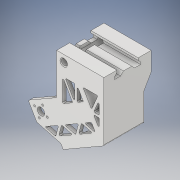
# Autodesk Inventor part: Gantry_Mount
Saved by Autodesk Inventor 2019 (Build 230136000, 136)
## iProperties
Created: 2021-01-31
Part Number: Gantry_Mount
Material: ABS Plastic
Document SubType Name: Modeling
Designer: zhanb
Density: 1.06 g/cm^3
Appearance: Smooth - White
Author: zhanb
Autodesk Inventor part; units mm, degrees
ref_plane "YZ Plane" through (0, 0, 0) normal (1, 0, 0) x (0, 1, 0)
ref_plane "XZ Plane" through (0, 0, 0) normal (0, 1, 0) x (-1, 0, 0)
ref_plane "XY Plane" through (0, 0, 0) normal (0, 0, 1) x (1, 0, 0)
sketch "Sketch1" plane through (0, 0, 0) normal (0, 0, 1) x (1, 0, 0)
  line L0 (-25.4, -44.45) -> (-18.594091, -44.45)
  line L1 (25.4, -44.45) -> (25.4, -19.05) construction
  line L2 (25.4, 44.45) -> (-25.4, 44.45)
  line L3 (-25.4, 44.45) -> (-25.4, -42.513515)
  line L4 (-25.4, -44.45) -> (25.4, 44.45) construction
  line L5 (25.4, -44.45) -> (-25.4, 44.45) construction
  line L6 (-18.594091, -44.45) -> (25.4, -19.05)
  line L7 (-18.594091, -44.45) -> (-35.091874, -53.975) construction
  line L8 (-35.091874, -53.975) -> (-37.631874, -49.575591) construction
  line L9 (-37.631874, -49.575591) -> (-25.4, -42.513515) construction
  line L10 (-21.134091, -40.050591) -> (-18.594091, -44.45) construction
  line L11 (-18.594091, -44.45) -> (25.4, -44.45) construction
  line L12 (-25.4, -42.513515) -> (-25.4, -44.45)
  line L13 (-25.4, -42.513515) -> (-21.134091, -40.050591) construction
  line L14 (25.4, -19.05) -> (25.4, 44.45)
  point P0 (0, 0)
  dimension "d0" = 30
  dimension "d1" = 50.8
  dimension "d2" = 88.9
  dimension "d3" = 50.8
  dimension "d4" = 5.08
  dimension "d5" = 19.05
  constraints: 30 end point, 9 parallel, 5 perpendicular, 2 horizontal, 2 midpoint, 1 point on line
  measures "d0" angle of L0 L6
  measures "d1" distance of L0.end L1.end
  measures "d2" distance of L2.end L0.start
  measures "d3" distance of L2.start L2.end
  measures "d4" distance of L7.end L8.end
  measures "d5" distance of L0.end L7.end
extrude "Extrusion1" add sketch "Sketch1" along normal mid plane 50.8
sketch "Sketch5" plane through (-25.4, -42.513515, 25.4) normal (-1, 0, 0) x (0, 0, 1)
  line L0 (0, 86.963515) -> (0, -1.936485) construction
  line L1 (-50.8, 86.963515) -> (0, 86.963515) construction
  line L2 (-50.8, -1.936485) -> (-50.8, 86.963515) construction
  line L3 (-36.83, 86.963515) -> (-36.83, 84.621952)
  line L4 (-36.83, 84.621952) -> (-39.37, 82.081952)
  line L5 (-39.37, 82.081952) -> (-39.37, 79.541952)
  line L6 (-39.37, 79.541952) -> (-33.02, 79.541952)
  line L7 (-33.02, 79.541952) -> (-29.845, 82.716952)
  line L8 (-29.845, 82.716952) -> (-20.955, 82.716952)
  line L9 (-20.955, 82.716952) -> (-17.78, 79.541952)
  line L10 (-17.78, 79.541952) -> (-11.43, 79.541952)
  line L11 (-11.43, 79.541952) -> (-11.43, 82.081952)
  line L12 (-11.43, 82.081952) -> (-13.97, 84.621952)
  line L13 (-13.97, 84.621952) -> (-13.97, 86.963515)
  line L14 (-25.4, 42.513515) -> (-25.4, 86.963515) construction
  line L15 (-36.83, 86.963515) -> (-13.97, 86.963515)
  line L16 (0, -1.936485) -> (-50.8, -1.936485)
  point P0 (-25.4, 42.513515)
  dimension "d22" = 135
  dimension "d23" = 11.43
  dimension "d24" = 2.34156
  dimension "d25" = 2.54
  dimension "d26" = 3.175
  dimension "d27" = 13.97
  dimension "d28" = 6.35
  constraints: 26 end point, 4 parallel, 4 point on line, 2 perpendicular, 1 coincident, 1 collinear, 1 midpoint, 5 other
  measures "d22" angle of L7 L8
  measures "d23" distance between parallel lines of L14 L3
  measures "d24" distance of L3.start L3.end
  measures "d25" distance of L4.end L5.end
  measures "d26" distance between parallel lines of L6 L8
  measures "d27" distance between parallel lines of L14 L5
  measures "d28" distance of L5.end L6.end
extrude "Extrusion3" cut sketch "Sketch5" against normal through all
sketch "Sketch6" plane through (0, 0, 25.4) normal (0, 0, 1) x (1, 0, 0)
  line L0 (-25.4, 37.028437) -> (25.4, 37.028437) construction
  line L1 (-25.4, 37.028437) -> (25.4, 37.028437) construction
  circle A0 centre (-17.78, 36.939538) radius 3.2639
  line L2 (-25.4, 44.45) -> (-25.4, -44.45)
  line L3 (25.4, 44.45) -> (-25.4, 44.45)
  line L4 (-25.4, 40.203438) -> (25.4, 40.203438) construction
  point P0 (0, 0)
  point P1 (0, 37.028437)
  point P2 (-25.4, -42.513515)
  dimension "d32" = 6.5278
  dimension "d35" = 7.62
  dimension "d39" = 3.2639
  constraints: 1 centre point, 1 coincident, 1 midpoint
  measures "d32" diameter of A0
  measures "d35" distance from line of L2 A0.centre
  measures "d39" distance from line of L4 point (-17.78, 36.94)
extrude "Extrusion4" cut sketch "Sketch6" against normal through all
sketch "Sketch7" plane through (0, 0, 0) normal (0, 0, 1) x (1, 0, 0)
  circle A0 centre (-17.78, 36.939538) radius 3.2639 construction
  arc A1 (-19.714406, 39.568437) -> (-21.042689, 37.028437) centre (-17.78, 36.939538) ccw construction
  line L0 (-21.0439, 36.939538) -> (-21.0439, 40.203438)
  line L1 (-21.0439, 40.203438) -> (-14.5161, 40.203438)
  line L2 (-14.5161, 40.203438) -> (-14.5161, 36.939538)
  arc A2 (-21.042689, 37.028437) -> (-15.845594, 39.568437) centre (-17.78, 36.939538) ccw construction
  arc A3 (-21.0439, 36.939538) -> (-14.5161, 36.939538) centre (-17.78, 36.939538) ccw
  point P0 (0, 0)
  point P1 (-25.4, 40.203438)
  constraints: 6 end point, 4 point on circle, 3 tangent, 1 centre point, 1 coincident, 1 horizontal alignment, 1 parallel, 1 perpendicular, 1 vertical
extrude "Extrusion5" cut sketch "Sketch7" along normal up to surface (22.86 mm away) from surface at -11.43
sketch "Sketch9" plane through (0, 0, 0) normal (0, 0, 1) x (1, 0, 0)
  line L0 (-25.4, -44.45) -> (-25.4, 44.45) construction
  line L1 (-18.594091, -44.45) -> (-25.4, -44.45) construction
  line L2 (25.4, -19.05) -> (-18.594091, -44.45) construction
  line L3 (25.4, 44.45) -> (25.4, -19.05) construction
  line L4 (-18.38446, -44.32897) -> (-20.92446, -39.929561)
  line L5 (-20.92446, -39.929561) -> (20.32, -16.117061)
  line L6 (20.32, -16.117061) -> (9.906, 1.920516)
  line L7 (9.906, 1.920516) -> (-20.339937, -15.541984)
  line L8 (-20.339937, -15.541984) -> (-22.879937, -11.142574)
  line L9 (-22.879937, -11.142574) -> (7.366, 6.319926)
  line L10 (7.366, 6.319926) -> (20.32, 13.798921) construction
  line L11 (-3.031219, 24.328437) -> (-19.297796, 24.328437)
  line L12 (-25.4, 24.328437) -> (-25.4, -44.45)
  line L13 (-25.4, -44.45) -> (-18.594091, -44.45)
  line L14 (20.32, -16.117061) -> (20.32, 24.328437) construction
  line L15 (20.32, 24.328437) -> (-3.031219, 24.328437) construction
  line L16 (7.366, 6.319926) -> (-3.031219, 24.328437)
  line L17 (-21.0439, 37.028437) -> (-21.042689, 37.028437)
  line L18 (-25.4, 37.028437) -> (-21.042689, 37.028437) construction
  line L19 (-25.4, 37.028437) -> (-21.0439, 37.028437)
  line L20 (-18.174426, -6.592759) -> (-1.092926, -36.178785) construction
  line L21 (-1.092926, -36.178785) -> (18.154489, -25.066285) construction
  line L22 (18.154489, -25.066285) -> (1.072989, 4.519741) construction
  line L23 (1.072989, 4.519741) -> (-18.174426, -6.592759) construction
  line L24 (-18.174426, -6.592759) -> (18.154489, -25.066285) construction
  line L25 (-1.092926, -36.178785) -> (1.072989, 4.519741) construction
  line L26 (-18.594091, -44.45) -> (-18.38446, -44.32897)
  line L27 (-19.297796, 24.328437) -> (-25.4, 34.897765)
  line L28 (-25.4, 34.897765) -> (-25.4, 24.328437)
  line L29 (-25.4, 44.45) -> (-25.4, -44.45) construction
  line L30 (-19.297796, 24.328437) -> (-25.4, 24.328437) construction
  circle A0 centre (-17.78, 36.939538) radius 3.2639 construction
  circle A1 centre (-17.78, 36.939538) radius 7.62 construction
  line L31 (20.32, -5.957061) -> (14.305409, 4.460516)
  line L32 (14.305409, 4.460516) -> (20.32, 4.460516)
  line L33 (20.32, -5.957061) -> (20.32, 4.460516)
  line L34 (20.32, 21.029283) -> (20.32, 7.000516)
  line L35 (20.32, 7.000516) -> (14.468763, 7.000516)
  line L36 (14.468763, 7.000516) -> (20.32, 21.029283)
  line L37 (18.943961, 24.328437) -> (12.187382, 8.129048)
  line L38 (12.187382, 8.129048) -> (2.83466, 24.328437)
  line L39 (18.943961, 24.328437) -> (2.83466, 24.328437)
  line L40 (15.565671, 16.228743) -> (17.909935, 15.250977) construction
  line L41 (17.394382, 7.000516) -> (17.394382, 4.460516) construction
  line L42 (14.305409, 4.460516) -> (12.187382, 8.129048) construction
  line L43 (14.468763, 7.000516) -> (12.187382, 8.129048) construction
  line L44 (14.468763, 7.000516) -> (14.305409, 4.460516) construction
  line L45 (14.468763, 7.000516) -> (13.246395, 6.294782) construction
  line L46 (13.328072, 7.564782) -> (16.737803, 15.73986) construction
  line L47 (16.737803, 15.73986) -> (20.32, 24.328437) construction
  point P0 (0, 0)
  point P1 (-0.009969, -15.829522)
  dimension "d51" = 5.08
  dimension "d52" = 5.08
  dimension "d53" = 5.08
  dimension "d54" = 20.828
  dimension "d55" = 12.7
  dimension "d56" = 22.225
  dimension "d57" = 1.5875
  dimension "d58" = 1.5875
  dimension "d59" = 6.35
  dimension "d60" = 19.05
  dimension "d108" = 2.54
  dimension "d109" = 5.08
  dimension "d112" = 12.7
  constraints: 81 end point, 14 point on line, 12 perpendicular, 7 midpoint, 6 collinear, 6 parallel, 3 horizontal, 3 vertical, 2 tangent, 1 centre point, 1 coincident, 1 equal length, 1 other
  measures "d51" distance between parallel lines of L2 L5
  measures "d52" distance between parallel lines of L9 L7
  measures "d53" distance between parallel lines of L3 L14
  measures "d54" distance between parallel lines of L5 L7
  measures "d55" distance between parallel lines of L11 L18
  measures "d56" distance of L20.end L21.end
  measures "d57" distance between parallel lines of L9 L23
  measures "d58" distance between parallel lines of L2 L21
  measures "d59" distance between parallel lines of L6 L22
  measures "d60" distance between parallel lines of L20 L4
  measures "d108" distance between parallel lines of L35 L32
  measures "d109" distance between parallel lines of L6 L31
  measures "d112" distance between parallel lines of L4 L8
extrude "Extrusion8" cut sketch "Sketch9" along normal through all both and the other way through all
sketch "Sketch10" plane through (25.4, -19.05, -25.4) normal (0.5, -0.8660254, 0) x (0.8660254, 0.5, 0)
  circle A0 centre (-20.395439, 25.4) radius 11.1379
  line L0 (-50.557939, 0) -> (-2.932939, 0)
  line L1 (-2.932939, 0) -> (-37.857939, 0)
  point P0 (-12.472045, 25.4)
  point P1 (-26.745439, 0)
  point P2 (-20.395439, 0)
  dimension "d63" = 22.2758
  constraints: 2 midpoint, 1 centre point, 1 horizontal alignment, 1 vertical alignment
  measures "d63" diameter of A0
extrude "Extrusion9" cut sketch "Sketch10" against normal up to surface (30.988 mm away)
sketch "Sketch11" plane through (0, 0, 25.4) normal (0, 0, 1) x (1, 0, 0)
  line L0 (-18.38446, -44.32897) -> (25.4, -19.05) construction
  line L1 (25.4, -19.05) -> (25.4, 44.45) construction
  line L2 (25.4, 44.45) -> (-25.4, 44.45) construction
  line L3 (-25.4, 44.45) -> (-25.4, 34.897765) construction
  circle A0 centre (-17.78, 36.939538) radius 3.2639 construction
  line L4 (-22.879937, -11.142574) -> (-20.339937, -15.541984) construction
  line L5 (7.366, 6.319926) -> (-3.031219, 24.328437)
  line L6 (-55.904888, -17.161714) -> (-25.4, 0.450291)
  line L7 (-25.4, 0.450291) -> (-25.4, 34.897765)
  line L8 (-44.015732, -27.594337) -> (-48.965479, -19.021123) construction
  line L9 (-48.965479, -19.021123) -> (-40.392265, -14.071376) construction
  line L10 (-40.392265, -14.071376) -> (-35.442517, -22.64459) construction
  line L11 (-35.442517, -22.64459) -> (-44.015732, -27.594337) construction
  line L12 (-44.015732, -27.594337) -> (-40.392265, -14.071376) construction
  line L13 (-48.965479, -19.021123) -> (-35.442517, -22.64459) construction
  circle A1 centre (-42.203998, -20.832857) radius 4
  line L14 (-55.904888, -17.161714) -> (-46.756022, -33.008014)
  line L15 (-46.756022, -33.008014) -> (-20.92446, -39.929561)
  line L16 (-20.92446, -39.929561) -> (-18.38446, -44.32897) construction
  line L17 (-25.4, 34.897765) -> (-19.297796, 24.328437)
  line L18 (-19.297796, 24.328437) -> (-3.031219, 24.328437)
  line L19 (-3.031219, 24.328437) -> (7.366, 6.319926)
  line L20 (7.366, 6.319926) -> (-22.879937, -11.142574)
  line L21 (-22.879937, -11.142574) -> (-20.339937, -15.541984)
  line L22 (-20.339937, -15.541984) -> (9.906, 1.920516)
  line L23 (9.906, 1.920516) -> (20.32, -16.117061)
  line L24 (20.32, -16.117061) -> (-20.92446, -39.929561)
  line L25 (7.366, 6.319926) -> (-22.879937, -11.142574)
  line L26 (-22.879937, -11.142574) -> (-20.339937, -15.541984)
  line L27 (9.906, 1.920516) -> (20.32, -16.117061)
  line L28 (-20.339937, -15.541984) -> (9.906, 1.920516)
  line L29 (20.32, -16.117061) -> (-20.92446, -39.929561)
  line L30 (-19.297796, 24.328437) -> (-25.4, 34.897765)
  line L31 (-25.4, 34.897765) -> (-19.297796, 24.328437)
  line L32 (-19.297796, 24.328437) -> (-3.031219, 24.328437)
  line L33 (-19.297796, 24.328437) -> (-3.031219, 24.328437)
  line L34 (-3.031219, 24.328437) -> (7.366, 6.319926)
  line L35 (7.366, 6.319926) -> (9.906, 1.920516)
  point P0 (0, 0)
  point P1 (0, 0)
  dimension "d86" = 8
  dimension "d87" = 14
  dimension "d90" = 5.08
  dimension "d104" = 5.08
  dimension "d110" = 45
  dimension "d114" = 6.35
  dimension "d115" = 42.418
  constraints: 36 end point, 6 parallel, 5 coincident, 3 collinear, 3 perpendicular, 2 midpoint, 1 centre point, 1 vertical
  measures "d86" diameter of A1
  measures "d87" distance of L8.start L9.end
  measures "d90" distance between parallel lines of L6 L9
  measures "d104" distance between parallel lines of L8 L14
  measures "d110" angle of L14 L15
  measures "d114" distance from line of L22 point (-42.204, -20.833)
  measures "d115" distance from line of L17 point (-42.204, -20.833)
extrude "Extrusion10" add sketch "Sketch11" against normal blind 3.81
hole "Hole3" at (-35.442517, -22.64459, 25.4) at (-44.015732, -27.594337, 25.4) at (-48.965479, -19.021123, 25.4) at (-40.392265, -14.071376, 25.4) direction (0, 0, -1) diameter 2.1 end through all both
chamfer "Chamfer1" distance 4.7625 angle 45 7 edges at (20.32, -16.1171, -1.905) (-0.3022, -28.0233, 21.59) (7.366, 6.3199, -1.905) (-7.757, -2.4113, 21.59) (-5.217, -6.8107, 21.59) (9.906, 1.9205, -1.905) (-21.6099, -13.3423, 21.59)
sketch "Sketch16" plane through (25.4, -19.05, 25.4) normal (1, 0, 0) x (0, 0, -1)
  line L0 (50.8, 43.378437) -> (50.8, 53.947765) construction
  line L1 (50.8, 43.378437) -> (42.8625, 29.494372)
  line L2 (3.81, 29.494372) -> (50.8, 29.494372) construction
  line L3 (42.8625, 29.494372) -> (42.8625, -25.27897)
  line L4 (0, -25.27897) -> (50.8, -25.27897) construction
  line L5 (42.8625, -25.27897) -> (50.8, -25.27897)
  line L6 (50.8, 29.494372) -> (50.8, 43.378437)
  line L7 (50.8, -25.27897) -> (50.8, 43.378437)
  point P0 (25.4, 19.05)
  dimension "d116" = 7.9375
  constraints: 8 end point, 1 collinear, 1 perpendicular, 1 point on line, 1 vertical
  measures "d116" distance between parallel lines of L7 L3
extrude "Extrusion14" cut sketch "Sketch16" against normal through all
fillet "Fillet1" radius 17.4752 1 edges at (-21.6099, -13.3423, -17.4625)
sketch "Sketch17" plane through (-20.92446, -39.929561, 16.8275) normal (-0.5, 0.8660254, 0) x (0.8660254, 0.5, 0)
  arc A0 (30.1752, 34.29) -> (12.7, 16.8148) centre (30.1752, 16.8148) ccw construction
  line L0 (0, 0) -> (0, 34.29)
  line L1 (15.115224, 25.679322) -> (0, 0)
  arc A1 (30.1752, 34.29) -> (15.115224, 25.679322) centre (30.1752, 16.8148) ccw
  line L2 (42.8625, 34.29) -> (0, 34.29)
  line L3 (30.1752, 34.29) -> (0, 34.29)
  line L4 (0, 34.29) -> (0, 0)
  point P0 (38.085894, 16.8275)
  constraints: 6 end point, 3 point on circle, 2 tangent, 1 centre point, 1 coincident, 1 collinear, 1 perpendicular
extrude "Extrusion15" cut sketch "Sketch17" against normal up to surface (5.08 mm away)
sketch "Sketch18" plane through (0, 0, 21.59) normal (0, 0, -1) x (-1, 0, 0)
  line L0 (-12.28725, -2.20393) -> (22.083133, -22.04768) construction
  line L1 (-17.93875, -11.992615) -> (-12.28725, -2.20393) construction
  line L2 (27.430156, -38.186365) -> (-17.93875, -11.992615) construction
  line L3 (27.430156, -38.186365) -> (46.756022, -33.008014) construction
  line L4 (46.756022, -33.008014) -> (55.904888, -17.161714) construction
  line L5 (55.904888, -17.161714) -> (25.4, 0.450291) construction
  line L6 (25.4, 0.450291) -> (25.4, 34.897765) construction
  line L7 (19.297796, 24.328437) -> (25.4, 34.897765) construction
  line L8 (3.031219, 24.328437) -> (19.297796, 24.328437) construction
  line L9 (-4.98475, 10.444372) -> (3.031219, 24.328437) construction
  line L10 (29.385633, -9.399378) -> (-4.98475, 10.444372) construction
  line L11 (22.083133, -22.04768) -> (29.385633, -9.399378) construction
  circle A0 centre (42.203998, -20.832857) radius 4 construction
  circle A1 centre (40.392265, -14.071376) radius 1.05 construction
  circle A2 centre (44.015732, -27.594337) radius 1.05 construction
  circle A3 centre (35.442517, -22.64459) radius 1.05 construction
  circle A4 centre (48.965479, -19.021123) radius 1.05 construction
  line L12 (-3.469868, 11.036224) -> (3.364572, 22.873821)
  line L13 (3.364572, 22.873821) -> (3.364572, 7.090358)
  line L14 (3.364572, 7.090358) -> (-3.469868, 11.036224)
  line L15 (5.904572, 23.312437) -> (5.904572, 5.623888)
  line L16 (5.904572, 5.623888) -> (16.117061, 23.312437)
  line L17 (16.117061, 23.312437) -> (5.904572, 23.312437)
  line L18 (19.05, 23.312437) -> (8.104276, 4.353888)
  line L19 (8.104276, 4.353888) -> (19.05, -1.965628)
  line L20 (19.05, -1.965628) -> (19.05, 23.312437)
  line L21 (-12.042368, -3.811782) -> (-16.423868, -11.400762)
  line L22 (-16.423868, -11.400762) -> (-4.453388, -8.193282)
  line L23 (-4.453388, -8.193282) -> (-12.042368, -3.811782)
  line L24 (-13.313016, -13.196814) -> (-1.342536, -9.989333)
  line L25 (-1.342536, -9.989333) -> (1.864945, -21.959814)
  line L26 (1.864945, -21.959814) -> (-13.313016, -13.196814)
  line L27 (1.768316, -11.785384) -> (4.975797, -23.755865)
  line L28 (4.975797, -23.755865) -> (16.946278, -20.548384)
  line L29 (16.946278, -20.548384) -> (1.768316, -11.785384)
  line L30 (8.086649, -25.551916) -> (20.05713, -22.344435)
  line L31 (20.05713, -22.344435) -> (23.26461, -34.314916)
  line L32 (23.26461, -34.314916) -> (8.086649, -25.551916)
  line L33 (25.4, 0.450291) -> (25.4, 34.897765) construction
  line L34 (-4.98475, 10.444372) -> (3.031219, 24.328437) construction
  line L35 (29.385633, -9.399378) -> (-4.98475, 10.444372) construction
  line L36 (3.031219, 24.328437) -> (19.297796, 24.328437) construction
  line L37 (-12.28725, -2.20393) -> (22.083133, -22.04768) construction
  line L38 (27.430156, -38.186365) -> (-17.93875, -11.992615) construction
  line L39 (-5.724036, -17.578314) -> (-1.342536, -9.989333) construction
  line L40 (15.67563, -29.933416) -> (20.05713, -22.344435) construction
  line L41 (4.975797, -23.755865) -> (9.357297, -16.166884) construction
  line L42 (1.864945, -21.959814) -> (4.975797, -23.755865) construction
  line L43 (4.975797, -23.755865) -> (8.086649, -25.551916) construction
  line L44 (-13.313016, -13.196814) -> (-16.423868, -11.400762) construction
  line L45 (23.167982, -24.140487) -> (26.375462, -36.110967)
  line L46 (26.375462, -36.110967) -> (38.345943, -32.903487)
  line L47 (38.345943, -32.903487) -> (30.756962, -28.521987)
  line L48 (26.375462, -36.110967) -> (30.756962, -28.521987) construction
  line L49 (23.26461, -34.314916) -> (26.375462, -36.110967) construction
  line L50 (30.756962, -28.521987) -> (23.167982, -24.140487)
  line L51 (3.364572, 7.090358) -> (5.904572, 7.090358) construction
  line L52 (5.904572, 5.623888) -> (8.104276, 4.353888) construction
  line L53 (19.297796, 24.328437) -> (25.4, 34.897765)
  point P0 (0, 0)
  dimension "d122" = 1.016
  dimension "d123" = 1.27
  dimension "d124" = 1.27
  dimension "d125" = 1.27
  dimension "d126" = 2.54
  dimension "d127" = 45
  dimension "d128" = 2.54
  dimension "d129" = 1.016
  dimension "d131" = 6.35
  constraints: 70 end point, 18 parallel, 10 collinear, 6 point on line, 5 equal length, 3 midpoint, 1 horizontal, 1 perpendicular, 1 other
  measures "d122" distance between parallel lines of L9 L12
  measures "d123" distance between parallel lines of L10 L14
  measures "d124" distance between parallel lines of L0 L23
  measures "d125" distance between parallel lines of L2 L26
  measures "d126" distance between parallel lines of L24 L22
  measures "d127" angle of L39 L25
  measures "d128" distance between parallel lines of L13 L15
  measures "d129" distance between parallel lines of L8 L17
  measures "d131" distance between parallel lines of L6 L20
extrude "Extrusion16" cut sketch "Sketch18" against normal up to surface (3.81 mm away)
fillet "Fillet2" radius 0.79375 24 edges at (-5.9046, 23.3124, 23.495) (-5.9046, 5.6239, 23.495) (-16.1171, 23.3124, 23.495) (-19.05, -1.9656, 23.495) (-19.05, 23.3124, 23.495) (-8.1043, 4.3539, 23.495) (1.3425, -9.9893, 23.495) (13.313, -13.1968, 23.495) (-1.8649, -21.9598, 23.495) (-23.2646, -34.3149, 23.495) (-20.0571, -22.3444, 23.495) (-8.0866, -25.5519, 23.495) (-3.3646, 22.8738, 23.495) (3.4699, 11.0362, 23.495) (-3.3646, 7.0904, 23.495) (4.4534, -8.1933, 23.495) (12.0424, -3.8118, 23.495) (16.4239, -11.4008, 23.495) (-26.3755, -36.111, 23.495) (-38.3459, -32.9035, 23.495) (-23.168, -24.1405, 23.495) (-16.9463, -20.5484, 23.495) (-1.7683, -11.7854, 23.495) (-4.9758, -23.7559, 23.495)
fillet "Fillet2" radius 0.79375 9 edges at (2.8347, 24.3284, 0) (18.944, 24.3284, 0) (12.1874, 8.129, 3.9688) (14.4688, 7.0005, 3.9687) (20.32, 21.0293, 0.9431) (20.32, 7.0005, 3.9688) (14.3054, 4.4605, 3.9688) (20.32, 4.4605, 3.9687) (20.32, -5.9571, 3.9687)
fillet "Fillet3" radius 1.5875 14 edges at (-19.2978, 24.3284, -1.905) (-25.4, 34.8978, -1.905) (-3.0312, 24.3284, -1.905) (4.9847, 10.4444, 2.0637) (12.2872, -2.2039, 2.0637) (17.9387, -11.9926, 2.0637) (5.7816, -0.4607, -0.3175) (16.1956, -18.4983, -0.3175) (3.2416, 3.9387, -0.3175) (25.4, -19.05, 3.9687) (-25.4, 0.4503, 23.495) (-55.9049, -17.1617, 23.495) (-46.756, -33.008, 23.495) (-20.9245, -39.9296, 21.1138)
chamfer "Chamfer3" distance 0.79375 angle 45 2 edges at (-21.0439, 36.9395, 25.4) (-21.0439, 36.9395, -25.4)
equation "\"d39\" = 0.5 * d32"
equation "\"d52\" = d51"
equation "\"d53\" = d51"
equation "\"d90\" = d104"
body "Solid1"
